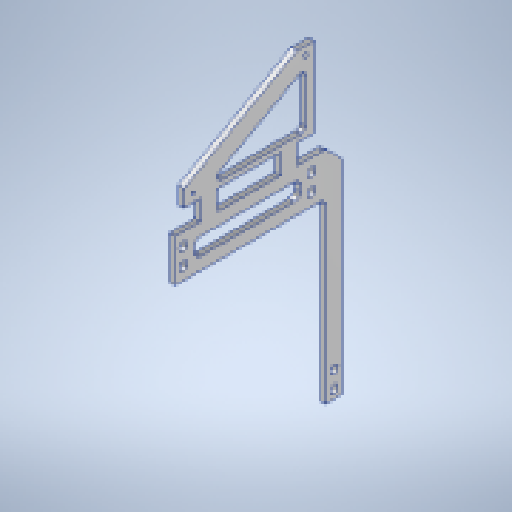
# Autodesk Inventor part: Swerve_v1_unit1_DRIVE_Plate_KaiseiMount
Saved by Autodesk Inventor 2025.4 (Build 294407020, 407B)
## iProperties
Created: 2026-08-26
Part Number: Swerve_v1_unit1_DRIVE_Plate_KaiseiMount
Material: アルミニウム 6061
Document SubType Name: Modeling
Designer: tanan
Density: 2.7 g/cm^3
Appearance: アルミニウム - フラット
Author: tanan
Autodesk Inventor part; units mm, degrees
ref_plane "YZ Plane" through (0, 0, 0) normal (1, 0, 0) x (0, 1, 0)
ref_plane "XZ Plane" through (0, 0, 0) normal (0, 1, 0) x (-1, 0, 0)
ref_plane "XY Plane" through (0, 0, 0) normal (0, 0, 1) x (1, 0, 0)
sketch "スケッチ1" plane through (0, 0, 0) normal (1, 0, 0) x (0, 1, 0)
  line L0 (0, 0) -> (15, 0)
  line L1 (15, 0) -> (15, -53)
  line L2 (15, -53) -> (0, -53)
  line L3 (0, -53) -> (0, 0)
  line L4 (9, -53) -> (-62.5, -53)
  line L5 (-62.5, -53) -> (-62.5, -59)
  line L6 (-62.5, -59) -> (9, -59)
  line L7 (9, -59) -> (9, -53)
  line L8 (15, -53) -> (9, -59)
  line L9 (0, -53) -> (0, -53)
  line L10 (10.5, -3) -> (4.5, -3)
  line L11 (4.5, -3) -> (4.5, -48)
  line L12 (4.5, -48) -> (10.5, -48)
  line L13 (10.5, -48) -> (10.5, -3)
  line L14 (15, -50.5) -> (0, -50.5)
  point P0 (7.5, 0)
  point P1 (7.5, -3)
  point P2 (-53.5, -56)
  point P3 (-59.5, -56)
  point P4 (-62.5, -56)
  dimension "d0" = 53
  dimension "d4" = 6
  dimension "d5" = 3
  dimension "d6" = 5
  dimension "d22" = 4.5
  dimension "d23" = 6
  dimension "d24" = 6
  dimension "d25" = 3
  dimension "d26" = 73
  dimension "d27" = 2.5
  dimension "d28" = 2.5
  dimension "d29" = 135
  constraints: 30 end point, 6 parallel, 4 horizontal, 4 perpendicular, 3 midpoint, 3 point on line, 2 horizontal alignment, 1 vertical alignment
  measures "d0" distance between parallel lines of L0 L2
  measures "d4" distance of L10.start L10.end
  measures "d5" distance from line of point (7.5, 0) L10
  measures "d6" distance between parallel lines of L2 L12
  measures "d22" distance between parallel lines of L3 L11
  measures "d23" distance of L4.end L5.end
  measures "d24" distance of point (-59.5, -56) point (-53.5, -56)
  measures "d25" distance from line of L5 point (-59.5, -56)
  measures "d26" distance between parallel lines of L5 L13
  measures "d27" distance between parallel lines of L12 L14
  measures "d28" distance between parallel lines of L14 L4
  measures "d29" angle of L1 L8
extrude "押し出し1" add sketch "スケッチ1" along normal blind 2 contours L0 L1 L14 L3 | L14 L1 L2 L3 | L2 L7 L6 L5 L4 | L8 L7 L2 | L13 L12 L11 L10
hole "穴1" at (0, 10.5, -3) at (0, 4.5, -3) at (0, 10.5, -48) at (0, 4.5, -48) at (0, -53.5, -56) at (0, -59.5, -56) direction (1, 0, 0) diameter 3 depth 8.8
sketch "スケッチ2" plane through (2, 0, 0) normal (1, 0, 0) x (0, 0, -1)
  line L0 (9, 10.5) -> (42, 10.5)
  line L1 (44, 8.5) -> (44, 6.5)
  line L2 (42, 4.5) -> (9, 4.5)
  line L3 (7, 6.5) -> (7, 8.5)
  line L4 (0, 15) -> (0, 0) projected
  circle A0 centre (3, 10.5) radius 1.5 projected
  circle A1 centre (48, 10.5) radius 1.5 projected
  arc A2 (9, 10.5) -> (7, 8.5) centre (9, 8.5) ccw
  arc A3 (7, 6.5) -> (9, 4.5) centre (9, 6.5) ccw
  arc A4 (42, 4.5) -> (44, 6.5) centre (42, 6.5) ccw
  arc A5 (44, 8.5) -> (42, 10.5) centre (42, 8.5) ccw
  point P0 (44, 10.5)
  point P1 (7, 7.5)
  point P2 (0, 7.5)
  dimension "d16" = 4
  dimension "d17" = 4
  dimension "d18" = 2
  constraints: 8 end point, 8 point on circle, 8 tangent, 4 centre point, 3 equal radius, 2 horizontal alignment, 2 midpoint, 2 parallel, 2 point on line, 1 horizontal, 1 perpendicular
  measures "d16" distance from line of L3 A0.centre
  measures "d17" distance from line of A1.centre L1
  measures "d18" radius of A2
extrude "押し出し2" cut sketch "スケッチ2" against normal blind 2 contours L0 A5 L1 A4 L2 A3 L3 A2
fillet "フィレット1" radius 2 1 edges at (1, 15, -53)
fillet "フィレット2" radius 2 2 edges at (1, 9, -59) (1, 0, -53)
sketch "スケッチ3" plane through (0, 0, 0) normal (-1, 0, 0) x (0, 0, 1)
  line L0 (-52.1716, 15) -> (0, 15) projected
  line L1 (-48.9108, 22) -> (-3.2608, 22)
  line L2 (-3.2608, 22) -> (-3.2608, 50.0429)
  line L3 (-3.2608, 50.0429) -> (-48.9108, 50.0429)
  line L4 (-48.9108, 50.0429) -> (-48.9108, 22)
  line L5 (-45.9108, 47.0429) -> (-6.2608, 25)
  line L6 (-52.1716, 15) -> (0, 15) projected
  line L7 (-42.9108, 50.0429) -> (-3.2608, 28)
  line L8 (-45.9108, 43.6105) -> (-45.9108, 24)
  line L9 (-45.9108, 24) -> (-10.6362, 24)
  line L10 (-10.6362, 24) -> (-45.9108, 43.6105)
  line L11 (-43.0858, 22) -> (-43.0858, 15)
  line L12 (-9.0858, 22) -> (-9.0858, 15)
  line L13 (-43.0858, 18.5) -> (-9.0858, 18.5)
  line L14 (-37.0858, 22) -> (-37.0858, 15)
  line L15 (-15.0858, 22) -> (-15.0858, 15)
  line L16 (-37.0858, 22) -> (-37.0858, 15)
  point P0 (0, 0)
  point P1 (-26.0858, 36.0215)
  point P2 (-26.0858, 15)
  point P3 (-3.2608, 15)
  point P4 (-26.0858, 18.5)
  point P5 (-26.0858, 15)
  point P6 (-9.0858, 15)
  point P7 (-15.0858, 18.5)
  point P8 (-37.0858, 18.5)
  point P9 (-37.0858, 18.5)
  dimension "d35" = 3
  dimension "d37" = 39.65
  dimension "d38" = 22.0429
  dimension "d39" = 3
  dimension "d40" = 3
  dimension "d41" = 3
  dimension "d44" = 10
  dimension "d45" = 3
  dimension "d46" = 3
  dimension "d47" = 2
  dimension "d56" = 3
  dimension "d57" = 34
  dimension "d58" = 6
  dimension "d59" = 6
  constraints: 30 end point, 6 perpendicular, 6 point on line, 5 midpoint, 4 parallel, 2 vertical, 2 vertical alignment, 1 horizontal, 6 other
  measures "d35" distance from line of L2 L5.end
  measures "d37" horizontal distance of L5.end L5.start
  measures "d38" vertical distance of L5.end L5.start
  measures "d39" distance from line of L4 L5.start
  measures "d40" distance from line of L3 L5.start
  measures "d41" horizontal distance of L5.start L7.start
  measures "d44" distance from line of L0 L5.end
  measures "d45" distance between parallel lines of L5 L10
  measures "d46" distance between parallel lines of L4 L8
  measures "d47" distance between parallel lines of L1 L9
  measures "d56" distance from line of L5.end L1
  measures "d57" distance between parallel lines of L12 L11
  measures "d58" distance between parallel lines of L11 L14
  measures "d59" distance between parallel lines of L12 L15
extrude "押し出し3" add sketch "スケッチ3" against normal blind 2 contours L11 L13 L14 L0 | L11 L1 L14 L13 | L15 L13 L12 L0 | L1 L4 L3 L7 L2 | L15 L1 L12 L13
hole "穴2" at (0, 47.0429, -45.9108) at (0, 25, -6.2608) direction (1, 0, 0) diameter 1.5 depth 13
fillet "フィレット3" radius 1.5 3 edges at (1, 43.6105, -45.9108) (1, 24, -10.6362) (1, 24, -45.9108)
fillet "フィレット4" radius 1.5 13 edges at (1, 15, -43.0858) (1, 22, -43.0858) (1, 22, -48.9108) (1, 22, -37.0858) (1, 15, -37.0858) (1, 15, -15.0858) (1, 22, -15.0858) (1, 22, -9.0858) (1, 22, -3.2608) (1, 15, -9.0858) (1, 28, -3.2608) (1, 50.0429, -48.9108) (1, 50.0429, -42.9108)
equation "\"d1\" = 1"
